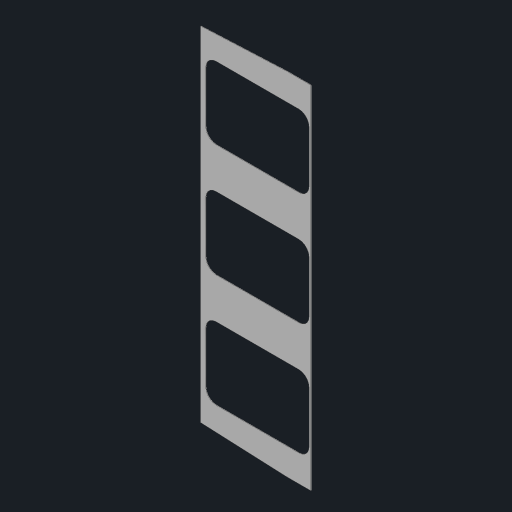
# Autodesk Inventor part: CARCASA_ALUM_5
Saved by Autodesk Inventor 2024.3 (Build 283343000, 343)
## iProperties
Created: 2024-05-15
Part Number: CARCASA_ALUM_5
Material: Generic
Document SubType Name: Sheet Metal
Designer: Niler
Density: 1 g/cm^3
Sheet Metal Rule: Default_mm
Appearance: Default
Author: Niler
Autodesk Inventor part; units mm, degrees
ref_plane "YZ Plane" through (0, 0, 0) normal (1, 0, 0) x (0, 1, 0)
ref_plane "XZ Plane" through (0, 0, 0) normal (0, 1, 0) x (-1, 0, 0)
ref_plane "Work Plane1" through (0, 0, 0) normal (0, 0, 1) x (1, 0, 0)
sketch "Sketch1" plane through (0, 0, 0) normal (0, 0, 1) x (1, 0, 0)
  arc A0 (535, 222.5775) -> (565, 252.5775) centre (535, 252.5775) ccw
  line L0 (535, 222.5775) -> (295, 222.5775)
  arc A1 (265, 252.5775) -> (295, 222.5775) centre (295, 252.5775) ccw
  line L1 (265, 252.5775) -> (265, 402.5775)
  arc A2 (295, 432.5775) -> (265, 402.5775) centre (295, 402.5775) ccw
  line L2 (295, 432.5775) -> (535, 432.5775)
  arc A3 (565, 402.5775) -> (535, 432.5775) centre (535, 402.5775) ccw
  line L3 (565, 402.5775) -> (565, 252.5775)
  arc A4 (535, -104.9225) -> (565, -74.9225) centre (535, -74.9225) ccw
  line L4 (535, -104.9225) -> (295, -104.9225)
  arc A5 (265, -74.9225) -> (295, -104.9225) centre (295, -74.9225) ccw
  line L5 (265, -74.9225) -> (265, 75.0775)
  arc A6 (295, 105.0775) -> (265, 75.0775) centre (295, 75.0775) ccw
  line L6 (295, 105.0775) -> (535, 105.0775)
  arc A7 (565, 75.0775) -> (535, 105.0775) centre (535, 75.0775) ccw
  line L7 (565, 75.0775) -> (565, -74.9225)
  line L8 (565, -252.4225) -> (565, -402.4225)
  arc A8 (535, -432.4225) -> (565, -402.4225) centre (535, -402.4225) ccw
  line L9 (535, -432.4225) -> (295, -432.4225)
  arc A9 (265, -402.4225) -> (295, -432.4225) centre (295, -402.4225) ccw
  line L10 (265, -402.4225) -> (265, -252.4225)
  arc A10 (295, -222.4225) -> (265, -252.4225) centre (295, -252.4225) ccw
  line L11 (295, -222.4225) -> (535, -222.4225)
  arc A11 (565, -252.4225) -> (535, -222.4225) centre (535, -252.4225) ccw
  line L12 (-550, 375.7749) -> (-550, 187.5)
  arc A12 (-473.6326, 455.6923) -> (-550, 375.7749) centre (-470, 375.7749) ccw
  line L13 (229.0918, 487.6344) -> (-473.6326, 455.6923)
  arc A13 (250, 467.655) -> (229.0918, 487.6344) centre (230, 467.655) ccw
  line L14 (250, 187.5) -> (250, 467.655)
  arc A14 (230, 167.5) -> (250, 187.5) centre (230, 187.5) ccw
  line L15 (-530, 167.5) -> (230, 167.5)
  arc A15 (-550, 187.5) -> (-530, 167.5) centre (-530, 187.5) ccw
  arc A16 (250, -187.5) -> (230, -167.5) centre (230, -187.5) ccw
  line L16 (250, -467.655) -> (250, -187.5)
  arc A17 (229.0918, -487.6344) -> (250, -467.655) centre (230, -467.655) ccw
  line L17 (-473.6326, -455.6923) -> (229.0918, -487.6344)
  arc A18 (-550, -375.7749) -> (-473.6326, -455.6923) centre (-470, -375.7749) ccw
  line L18 (-550, -187.5) -> (-550, -375.7749)
  arc A19 (-530, -167.5) -> (-550, -187.5) centre (-530, -187.5) ccw
  line L19 (230, -167.5) -> (-530, -167.5)
  line L20 (-550, 137.5) -> (-550, -137.5)
  arc A20 (-530, 157.5) -> (-550, 137.5) centre (-530, 137.5) ccw
  line L21 (230, 157.5) -> (-530, 157.5)
  arc A21 (250, 137.5) -> (230, 157.5) centre (230, 137.5) ccw
  line L22 (250, -137.5) -> (250, 137.5)
  arc A22 (230, -157.5) -> (250, -137.5) centre (230, -137.5) ccw
  line L23 (-530, -157.5) -> (230, -157.5)
  arc A23 (-550, -137.5) -> (-530, -157.5) centre (-530, -137.5) ccw
  line L24 (570.1484, 510) -> (570.1484, -510)
  line L25 (500.9086, 510) -> (570.1484, 510)
  line L26 (-474.4993, 465.6633) -> (500.9086, 510)
  arc A24 (-474.4993, 465.6633) -> (-559.5063, 385.1982) centre (-470, 375.7749) ccw
  line L27 (-570.7648, 375.1108) -> (-559.5063, 385.1982)
  line L28 (-600, 375.7749) -> (-570.7648, 375.1108)
  line L29 (-600, -375.7749) -> (-600, 375.7749)
  line L30 (-570.7648, -375.1108) -> (-600, -375.7749)
  line L31 (-559.5063, -385.1982) -> (-570.7648, -375.1108)
  arc A25 (-559.5063, -385.1982) -> (-474.4993, -465.6633) centre (-470, -375.7749) ccw
  line L32 (500.9086, -510) -> (-474.4993, -465.6633)
  line L33 (570.1484, -510) -> (500.9086, -510)
  line L34 (250, 498.5951) -> (250, -498.5951)
  point P0 (0, 0)
extrude "Plate1" add sketch "Sketch1" against normal blind 1.5 contours L34 L26 L25 L24 L33 L32 L16 L22 L14
equation "\"d0\" = Thickness"
equation "\"BendRadius\" = Thickness"
equation "\"BendReliefWidth\" = Thickness"
equation "\"BendReliefDepth\" = 0.5 * Thickness"
equation "\"CornerReliefSize\" = 4 * Thickness"
equation "\"MinimumRemnant\" = 2 * Thickness"
equation "\"TransitionRadius\" = BendRadius"
equation "\"JacobiRadiusSize\" = BendRadius"
equation "\"GapSize\" = Thickness"
equation "\"Thickness\" = 1.5"
body "Solid1"
